Autodesk Fusion 360 part; units mm, degrees
(part 3 of 5)
  line L868 (18.5, -98.5) -> (1.5, -98.5)
  line L869 (1.5, -98.5) -> (1.5, -81.5)
  line L870 (1.5, -81.5) -> (18.5, -81.5)
  line L871 (18.5, -81.5) -> (18.5, -98.5)
  line L872 (38.5, -98.5) -> (21.5, -98.5)
  line L873 (21.5, -98.5) -> (21.5, -81.5)
  line L874 (21.5, -81.5) -> (38.5, -81.5)
  line L875 (38.5, -81.5) -> (38.5, -98.5)
  line L876 (58.5, -98.5) -> (41.5, -98.5)
  line L877 (41.5, -98.5) -> (41.5, -81.5)
  line L878 (41.5, -81.5) -> (58.5, -81.5)
  line L879 (58.5, -81.5) -> (58.5, -98.5)
  line L880 (-105, -220) -> (105, -220)
  line L881 (105, -220) -> (105, 220)
  line L882 (105, 220) -> (-105, 220)
  line L883 (-105, 220) -> (-105, -220)
  line L884 (105, 220) -> (100, 220) construction
  line L885 (-105, 220) -> (-100, 220) construction
  line L886 (-100, 220) -> (-100, -220)
  line L887 (100, 220) -> (100, -220)
  dimension "d16" = 5
  dimension "d17" = 5
  constraint coincident L881.end L882.start
  constraint perpendicular L881 L884
  constraint coincident L882.end L883.start
  constraint perpendicular L883 L885
  constraint coincident L880 L886.end
  constraint perpendicular L880 L886
  constraint coincident L880 L887.end
  constraint perpendicular L880 L887
  measures "d16" distance of L881.end L884.end
  measures "d17" distance of L882.end L885.end
extrude "Extrude4" add sketch "Sketch2" along normal blind 1.6 contours L880 L882 L883 L886 | L880 L881 L882 L887 bodies 1
sketch "Sketch3" plane through (0, 0, 0) normal (0, 0, -1) x (-1, 0, 0)
  line L0 (-100, 220) -> (-100, -220)
  line L1 (-100, -220) -> (100, -220)
  line L2 (100, -220) -> (100, 220)
  line L3 (100, 220) -> (-100, 220)
  line L4 (58.5, -98.5) -> (41.5, -98.5)
  line L5 (41.5, -98.5) -> (41.5, -81.5)
  line L6 (41.5, -81.5) -> (58.5, -81.5)
  line L7 (58.5, -81.5) -> (58.5, -98.5)
  line L8 (38.5, -98.5) -> (21.5, -98.5)
  line L9 (21.5, -98.5) -> (21.5, -81.5)
  line L10 (21.5, -81.5) -> (38.5, -81.5)
  line L11 (38.5, -81.5) -> (38.5, -98.5)
  line L12 (18.5, -98.5) -> (1.5, -98.5)
  line L13 (1.5, -98.5) -> (1.5, -81.5)
  line L14 (1.5, -81.5) -> (18.5, -81.5)
  line L15 (18.5, -81.5) -> (18.5, -98.5)
  line L16 (-1.5, -98.5) -> (-18.5, -98.5)
  line L17 (-18.5, -98.5) -> (-18.5, -81.5)
  line L18 (-18.5, -81.5) -> (-1.5, -81.5)
  line L19 (-1.5, -81.5) -> (-1.5, -98.5)
  line L20 (-21.5, -98.5) -> (-38.5, -98.5)
  line L21 (-38.5, -98.5) -> (-38.5, -81.5)
  line L22 (-38.5, -81.5) -> (-21.5, -81.5)
  line L23 (-21.5, -81.5) -> (-21.5, -98.5)
  line L24 (-41.5, -98.5) -> (-58.5, -98.5)
  line L25 (-58.5, -98.5) -> (-58.5, -81.5)
  line L26 (-58.5, -81.5) -> (-41.5, -81.5)
  line L27 (-41.5, -81.5) -> (-41.5, -98.5)
  line L28 (-61.5, -98.5) -> (-78.5, -98.5)
  line L29 (-78.5, -98.5) -> (-78.5, -81.5)
  line L30 (-78.5, -81.5) -> (-61.5, -81.5)
  line L31 (-61.5, -81.5) -> (-61.5, -98.5)
  line L32 (-81.5, -98.5) -> (-98.5, -98.5)
  line L33 (-98.5, -98.5) -> (-98.5, -81.5)
  line L34 (-98.5, -81.5) -> (-81.5, -81.5)
  line L35 (-81.5, -81.5) -> (-81.5, -98.5)
  line L36 (98.5, -78.5) -> (81.5, -78.5)
  line L37 (81.5, -78.5) -> (81.5, -61.5)
  line L38 (81.5, -61.5) -> (98.5, -61.5)
  line L39 (98.5, -61.5) -> (98.5, -78.5)
  line L40 (78.5, -78.5) -> (61.5, -78.5)
  line L41 (61.5, -78.5) -> (61.5, -61.5)
  line L42 (61.5, -61.5) -> (78.5, -61.5)
  line L43 (78.5, -61.5) -> (78.5, -78.5)
  line L44 (58.5, -78.5) -> (41.5, -78.5)
  line L45 (41.5, -78.5) -> (41.5, -61.5)
  line L46 (41.5, -61.5) -> (58.5, -61.5)
  line L47 (58.5, -61.5) -> (58.5, -78.5)
  line L48 (38.5, -78.5) -> (21.5, -78.5)
  line L49 (21.5, -78.5) -> (21.5, -61.5)
  line L50 (21.5, -61.5) -> (38.5, -61.5)
  line L51 (38.5, -61.5) -> (38.5, -78.5)
  line L52 (18.5, -78.5) -> (1.5, -78.5)
  line L53 (1.5, -78.5) -> (1.5, -61.5)
  line L54 (1.5, -61.5) -> (18.5, -61.5)
  line L55 (18.5, -61.5) -> (18.5, -78.5)
  line L56 (-1.5, -78.5) -> (-18.5, -78.5)
  line L57 (-18.5, -78.5) -> (-18.5, -61.5)
  line L58 (-18.5, -61.5) -> (-1.5, -61.5)
  line L59 (-1.5, -61.5) -> (-1.5, -78.5)
  line L60 (-21.5, -78.5) -> (-38.5, -78.5)
  line L61 (-38.5, -78.5) -> (-38.5, -61.5)
  line L62 (-38.5, -61.5) -> (-21.5, -61.5)
  line L63 (-21.5, -61.5) -> (-21.5, -78.5)
  line L64 (-41.5, -78.5) -> (-58.5, -78.5)
  line L65 (-58.5, -78.5) -> (-58.5, -61.5)
  line L66 (-58.5, -61.5) -> (-41.5, -61.5)
  line L67 (-41.5, -61.5) -> (-41.5, -78.5)
  line L68 (-61.5, -78.5) -> (-78.5, -78.5)
  line L69 (-78.5, -78.5) -> (-78.5, -61.5)
  line L70 (-78.5, -61.5) -> (-61.5, -61.5)
  line L71 (-61.5, -61.5) -> (-61.5, -78.5)
  line L72 (-81.5, -78.5) -> (-98.5, -78.5)
  line L73 (-98.5, -78.5) -> (-98.5, -61.5)
  line L74 (-98.5, -61.5) -> (-81.5, -61.5)
  line L75 (-81.5, -61.5) -> (-81.5, -78.5)
  line L76 (98.5, -58.5) -> (81.5, -58.5)
  line L77 (81.5, -58.5) -> (81.5, -41.5)
  line L78 (81.5, -41.5) -> (98.5, -41.5)
  line L79 (98.5, -41.5) -> (98.5, -58.5)
  line L80 (78.5, -58.5) -> (61.5, -58.5)
  line L81 (61.5, -58.5) -> (61.5, -41.5)
  line L82 (61.5, -41.5) -> (78.5, -41.5)
  line L83 (78.5, -41.5) -> (78.5, -58.5)
  line L84 (58.5, -58.5) -> (41.5, -58.5)
  line L85 (41.5, -58.5) -> (41.5, -41.5)
  line L86 (41.5, -41.5) -> (58.5, -41.5)
  line L87 (58.5, -41.5) -> (58.5, -58.5)
  line L88 (38.5, -58.5) -> (21.5, -58.5)
  line L89 (21.5, -58.5) -> (21.5, -41.5)
  line L90 (21.5, -41.5) -> (38.5, -41.5)
  line L91 (38.5, -41.5) -> (38.5, -58.5)
  line L92 (18.5, -58.5) -> (1.5, -58.5)
  line L93 (1.5, -58.5) -> (1.5, -41.5)
  line L94 (1.5, -41.5) -> (18.5, -41.5)
  line L95 (18.5, -41.5) -> (18.5, -58.5)
  line L96 (-21.5, -58.5) -> (-38.5, -58.5)
  line L97 (-38.5, -58.5) -> (-38.5, -41.5)
  line L98 (-38.5, -41.5) -> (-21.5, -41.5)
  line L99 (-21.5, -41.5) -> (-21.5, -58.5)
  line L100 (78.5, 121.5) -> (61.5, 121.5)
  line L101 (61.5, 121.5) -> (61.5, 138.5)
  line L102 (61.5, 138.5) -> (78.5, 138.5)
  line L103 (78.5, 138.5) -> (78.5, 121.5)
  line L104 (18.5, 161.5) -> (1.5, 161.5)
  line L105 (1.5, 161.5) -> (1.5, 178.5)
  line L106 (1.5, 178.5) -> (18.5, 178.5)
  line L107 (18.5, 178.5) -> (18.5, 161.5)
  line L108 (-1.5, 161.5) -> (-18.5, 161.5)
  line L109 (-18.5, 161.5) -> (-18.5, 178.5)
  line L110 (-18.5, 178.5) -> (-1.5, 178.5)
  line L111 (-1.5, 178.5) -> (-1.5, 161.5)
  line L112 (-21.5, 161.5) -> (-38.5, 161.5)
  line L113 (-38.5, 161.5) -> (-38.5, 178.5)
  line L114 (-38.5, 178.5) -> (-21.5, 178.5)
  line L115 (-21.5, 178.5) -> (-21.5, 161.5)
  line L116 (-41.5, 161.5) -> (-58.5, 161.5)
  line L117 (-58.5, 161.5) -> (-58.5, 178.5)
  line L118 (-58.5, 178.5) -> (-41.5, 178.5)
  line L119 (-41.5, 178.5) -> (-41.5, 161.5)
  line L120 (-61.5, 161.5) -> (-78.5, 161.5)
  line L121 (-78.5, 161.5) -> (-78.5, 178.5)
  line L122 (-78.5, 178.5) -> (-61.5, 178.5)
  line L123 (-61.5, 178.5) -> (-61.5, 161.5)
  line L124 (-81.5, 161.5) -> (-98.5, 161.5)
  line L125 (-98.5, 161.5) -> (-98.5, 178.5)
  line L126 (-98.5, 178.5) -> (-81.5, 178.5)
  line L127 (-81.5, 178.5) -> (-81.5, 161.5)
  line L128 (98.5, 181.5) -> (81.5, 181.5)
  line L129 (81.5, 181.5) -> (81.5, 198.5)
  line L130 (81.5, 198.5) -> (98.5, 198.5)
  line L131 (98.5, 198.5) -> (98.5, 181.5)
  line L132 (78.5, 181.5) -> (61.5, 181.5)
  line L133 (61.5, 181.5) -> (61.5, 198.5)
  line L134 (61.5, 198.5) -> (78.5, 198.5)
  line L135 (78.5, 198.5) -> (78.5, 181.5)
  line L136 (58.5, 181.5) -> (41.5, 181.5)
  line L137 (41.5, 181.5) -> (41.5, 198.5)
  line L138 (41.5, 198.5) -> (58.5, 198.5)
  line L139 (58.5, 198.5) -> (58.5, 181.5)
  line L140 (38.5, 181.5) -> (21.5, 181.5)
  line L141 (21.5, 181.5) -> (21.5, 198.5)
  line L142 (21.5, 198.5) -> (38.5, 198.5)
  line L143 (38.5, 198.5) -> (38.5, 181.5)
  line L144 (18.5, 181.5) -> (1.5, 181.5)
  line L145 (1.5, 181.5) -> (1.5, 198.5)
  line L146 (1.5, 198.5) -> (18.5, 198.5)
  line L147 (18.5, 198.5) -> (18.5, 181.5)
  line L148 (-1.5, 181.5) -> (-18.5, 181.5)
  line L149 (-18.5, 181.5) -> (-18.5, 198.5)
  line L150 (-18.5, 198.5) -> (-1.5, 198.5)
  line L151 (-1.5, 198.5) -> (-1.5, 181.5)
  line L152 (-21.5, 181.5) -> (-38.5, 181.5)
  line L153 (-38.5, 181.5) -> (-38.5, 198.5)
  line L154 (-38.5, 198.5) -> (-21.5, 198.5)
  line L155 (-21.5, 198.5) -> (-21.5, 181.5)
  line L156 (-41.5, 181.5) -> (-58.5, 181.5)
  line L157 (-58.5, 181.5) -> (-58.5, 198.5)
  line L158 (-58.5, 198.5) -> (-41.5, 198.5)
  line L159 (-41.5, 198.5) -> (-41.5, 181.5)
  line L160 (-61.5, 181.5) -> (-78.5, 181.5)
  line L161 (-78.5, 181.5) -> (-78.5, 198.5)
  line L162 (-78.5, 198.5) -> (-61.5, 198.5)
  line L163 (-61.5, 198.5) -> (-61.5, 181.5)
  line L164 (-81.5, 181.5) -> (-98.5, 181.5)
  line L165 (-98.5, 181.5) -> (-98.5, 198.5)
  line L166 (-98.5, 198.5) -> (-81.5, 198.5)
  line L167 (-81.5, 198.5) -> (-81.5, 181.5)
  line L168 (98.5, 201.5) -> (81.5, 201.5)
  line L169 (81.5, 201.5) -> (81.5, 218.5)
  line L170 (81.5, 218.5) -> (98.5, 218.5)
  line L171 (98.5, 218.5) -> (98.5, 201.5)
  line L172 (78.5, 201.5) -> (61.5, 201.5)
  line L173 (61.5, 201.5) -> (61.5, 218.5)
  line L174 (61.5, 218.5) -> (78.5, 218.5)
  line L175 (78.5, 218.5) -> (78.5, 201.5)
  line L176 (58.5, 201.5) -> (41.5, 201.5)
  line L177 (41.5, 201.5) -> (41.5, 218.5)
  line L178 (41.5, 218.5) -> (58.5, 218.5)
  line L179 (58.5, 218.5) -> (58.5, 201.5)
  line L180 (38.5, 201.5) -> (21.5, 201.5)
  line L181 (21.5, 201.5) -> (21.5, 218.5)
  line L182 (21.5, 218.5) -> (38.5, 218.5)
  line L183 (38.5, 218.5) -> (38.5, 201.5)
  line L184 (18.5, 201.5) -> (1.5, 201.5)
  line L185 (1.5, 201.5) -> (1.5, 218.5)
  line L186 (1.5, 218.5) -> (18.5, 218.5)
  line L187 (18.5, 218.5) -> (18.5, 201.5)
  line L188 (-1.5, 201.5) -> (-18.5, 201.5)
  line L189 (-18.5, 201.5) -> (-18.5, 218.5)
  line L190 (-18.5, 218.5) -> (-1.5, 218.5)
  line L191 (-1.5, 218.5) -> (-1.5, 201.5)
  line L192 (-21.5, 201.5) -> (-38.5, 201.5)
  line L193 (-38.5, 201.5) -> (-38.5, 218.5)
  line L194 (-38.5, 218.5) -> (-21.5, 218.5)
  line L195 (-21.5, 218.5) -> (-21.5, 201.5)
  line L196 (-41.5, 201.5) -> (-58.5, 201.5)
  line L197 (-58.5, 201.5) -> (-58.5, 218.5)
  line L198 (-58.5, 218.5) -> (-41.5, 218.5)
  line L199 (-41.5, 218.5) -> (-41.5, 201.5)
  line L200 (-61.5, 201.5) -> (-78.5, 201.5)
  line L201 (-78.5, 201.5) -> (-78.5, 218.5)
  line L202 (-78.5, 218.5) -> (-61.5, 218.5)
  line L203 (-61.5, 218.5) -> (-61.5, 201.5)
  line L204 (-81.5, 201.5) -> (-98.5, 201.5)
  line L205 (-98.5, 201.5) -> (-98.5, 218.5)
  line L206 (-98.5, 218.5) -> (-81.5, 218.5)
  line L207 (-81.5, 218.5) -> (-81.5, 201.5)
  line L208 (-61.5, -58.5) -> (-78.5, -58.5)
  line L209 (-78.5, -58.5) -> (-78.5, -41.5)
  line L210 (-78.5, -41.5) -> (-61.5, -41.5)
  line L211 (-61.5, -41.5) -> (-61.5, -58.5)
  line L212 (-81.5, -58.5) -> (-98.5, -58.5)
  line L213 (-98.5, -58.5) -> (-98.5, -41.5)
  line L214 (-98.5, -41.5) -> (-81.5, -41.5)
  line L215 (-81.5, -41.5) -> (-81.5, -58.5)
  line L216 (98.5, -38.5) -> (81.5, -38.5)
  line L217 (81.5, -38.5) -> (81.5, -21.5)
  line L218 (81.5, -21.5) -> (98.5, -21.5)
  line L219 (98.5, -21.5) -> (98.5, -38.5)
  line L220 (78.5, -38.5) -> (61.5, -38.5)
  line L221 (61.5, -38.5) -> (61.5, -21.5)
  line L222 (61.5, -21.5) -> (78.5, -21.5)
  line L223 (78.5, -21.5) -> (78.5, -38.5)
  line L224 (58.5, -38.5) -> (41.5, -38.5)
  line L225 (41.5, -38.5) -> (41.5, -21.5)
  line L226 (41.5, -21.5) -> (58.5, -21.5)
  line L227 (58.5, -21.5) -> (58.5, -38.5)
  line L228 (38.5, -38.5) -> (21.5, -38.5)
  line L229 (21.5, -38.5) -> (21.5, -21.5)
  line L230 (21.5, -21.5) -> (38.5, -21.5)
  line L231 (38.5, -21.5) -> (38.5, -38.5)
  line L232 (18.5, -38.5) -> (1.5, -38.5)
  line L233 (1.5, -38.5) -> (1.5, -21.5)
  line L234 (1.5, -21.5) -> (18.5, -21.5)
  line L235 (18.5, -21.5) -> (18.5, -38.5)
  line L236 (-1.5, -38.5) -> (-18.5, -38.5)
  line L237 (-18.5, -38.5) -> (-18.5, -21.5)
  line L238 (-18.5, -21.5) -> (-1.5, -21.5)
  line L239 (-1.5, -21.5) -> (-1.5, -38.5)
  line L240 (-21.5, -38.5) -> (-38.5, -38.5)
  line L241 (-38.5, -38.5) -> (-38.5, -21.5)
  line L242 (-38.5, -21.5) -> (-21.5, -21.5)
  line L243 (-21.5, -21.5) -> (-21.5, -38.5)
  line L244 (-41.5, -38.5) -> (-58.5, -38.5)
  line L245 (-58.5, -38.5) -> (-58.5, -21.5)
  line L246 (-58.5, -21.5) -> (-41.5, -21.5)
  line L247 (-41.5, -21.5) -> (-41.5, -38.5)
  line L248 (-61.5, -38.5) -> (-78.5, -38.5)
  line L249 (-78.5, -38.5) -> (-78.5, -21.5)
  line L250 (-78.5, -21.5) -> (-61.5, -21.5)
  line L251 (-61.5, -21.5) -> (-61.5, -38.5)
  line L252 (-81.5, -38.5) -> (-98.5, -38.5)
  line L253 (-98.5, -38.5) -> (-98.5, -21.5)
  line L254 (-98.5, -21.5) -> (-81.5, -21.5)
  line L255 (-81.5, -21.5) -> (-81.5, -38.5)
  line L256 (98.5, -18.5) -> (81.5, -18.5)
  line L257 (81.5, -18.5) -> (81.5, -1.5)
  line L258 (81.5, -1.5) -> (98.5, -1.5)
  line L259 (98.5, -1.5) -> (98.5, -18.5)
  line L260 (78.5, -18.5) -> (61.5, -18.5)
  line L261 (61.5, -18.5) -> (61.5, -1.5)
  line L262 (61.5, -1.5) -> (78.5, -1.5)
  line L263 (78.5, -1.5) -> (78.5, -18.5)
  line L264 (58.5, -18.5) -> (41.5, -18.5)
  line L265 (41.5, -18.5) -> (41.5, -1.5)
  line L266 (41.5, -1.5) -> (58.5, -1.5)
  line L267 (58.5, -1.5) -> (58.5, -18.5)
  line L268 (38.5, -18.5) -> (21.5, -18.5)
  line L269 (21.5, -18.5) -> (21.5, -1.5)
  line L270 (21.5, -1.5) -> (38.5, -1.5)
  line L271 (38.5, -1.5) -> (38.5, -18.5)
  line L272 (18.5, -18.5) -> (1.5, -18.5)
  line L273 (1.5, -18.5) -> (1.5, -1.5)
  line L274 (1.5, -1.5) -> (18.5, -1.5)
  line L275 (18.5, -1.5) -> (18.5, -18.5)
  line L276 (-1.5, -18.5) -> (-18.5, -18.5)
  line L277 (-18.5, -18.5) -> (-18.5, -1.5)
  line L278 (-18.5, -1.5) -> (-1.5, -1.5)
  line L279 (-1.5, -1.5) -> (-1.5, -18.5)
  line L280 (-21.5, -18.5) -> (-38.5, -18.5)
  line L281 (-38.5, -18.5) -> (-38.5, -1.5)
  line L282 (-38.5, -1.5) -> (-21.5, -1.5)
  line L283 (-21.5, -1.5) -> (-21.5, -18.5)
  line L284 (-41.5, -18.5) -> (-58.5, -18.5)
  line L285 (-58.5, -18.5) -> (-58.5, -1.5)
  line L286 (-58.5, -1.5) -> (-41.5, -1.5)
  line L287 (-41.5, -1.5) -> (-41.5, -18.5)
  line L288 (-61.5, -18.5) -> (-78.5, -18.5)
  line L289 (-78.5, -18.5) -> (-78.5, -1.5)
  line L290 (-78.5, -1.5) -> (-61.5, -1.5)
  line L291 (-61.5, -1.5) -> (-61.5, -18.5)
  line L292 (-81.5, -18.5) -> (-98.5, -18.5)
  line L293 (-98.5, -18.5) -> (-98.5, -1.5)
  line L294 (-98.5, -1.5) -> (-81.5, -1.5)
  line L295 (-81.5, -1.5) -> (-81.5, -18.5)
  line L296 (98.5, 1.5) -> (81.5, 1.5)
  line L297 (81.5, 1.5) -> (81.5, 18.5)
  line L298 (81.5, 18.5) -> (98.5, 18.5)
  line L299 (98.5, 18.5) -> (98.5, 1.5)
  line L300 (78.5, 1.5) -> (61.5, 1.5)
  line L301 (61.5, 1.5) -> (61.5, 18.5)
  line L302 (61.5, 18.5) -> (78.5, 18.5)
  line L303 (78.5, 18.5) -> (78.5, 1.5)
  line L304 (58.5, 1.5) -> (41.5, 1.5)
  line L305 (41.5, 1.5) -> (41.5, 18.5)
  line L306 (41.5, 18.5) -> (58.5, 18.5)
  line L307 (58.5, 18.5) -> (58.5, 1.5)
  line L308 (38.5, 1.5) -> (21.5, 1.5)
  line L309 (21.5, 1.5) -> (21.5, 18.5)
  line L310 (21.5, 18.5) -> (38.5, 18.5)
  line L311 (38.5, 18.5) -> (38.5, 1.5)
  line L312 (18.5, 1.5) -> (1.5, 1.5)
  line L313 (1.5, 1.5) -> (1.5, 18.5)
  line L314 (1.5, 18.5) -> (18.5, 18.5)
  line L315 (18.5, 18.5) -> (18.5, 1.5)
  line L316 (-1.5, 1.5) -> (-18.5, 1.5)
  line L317 (-18.5, 1.5) -> (-18.5, 18.5)
  line L318 (-18.5, 18.5) -> (-1.5, 18.5)
  line L319 (-1.5, 18.5) -> (-1.5, 1.5)
  line L320 (-21.5, 1.5) -> (-38.5, 1.5)
  line L321 (-38.5, 1.5) -> (-38.5, 18.5)
  line L322 (-38.5, 18.5) -> (-21.5, 18.5)
  line L323 (-21.5, 18.5) -> (-21.5, 1.5)
  line L324 (-41.5, 1.5) -> (-58.5, 1.5)
  line L325 (-58.5, 1.5) -> (-58.5, 18.5)
  line L326 (-58.5, 18.5) -> (-41.5, 18.5)
  line L327 (-41.5, 18.5) -> (-41.5, 1.5)
  line L328 (-61.5, 1.5) -> (-78.5, 1.5)
  line L329 (-78.5, 1.5) -> (-78.5, 18.5)
  line L330 (-78.5, 18.5) -> (-61.5, 18.5)
  line L331 (-61.5, 18.5) -> (-61.5, 1.5)
  line L332 (-81.5, 1.5) -> (-98.5, 1.5)
  line L333 (-98.5, 1.5) -> (-98.5, 18.5)
  line L334 (-98.5, 18.5) -> (-81.5, 18.5)
  line L335 (-81.5, 18.5) -> (-81.5, 1.5)
  line L336 (98.5, 21.5) -> (81.5, 21.5)
  line L337 (81.5, 21.5) -> (81.5, 38.5)
  line L338 (81.5, 38.5) -> (98.5, 38.5)
  line L339 (98.5, 38.5) -> (98.5, 21.5)
  line L340 (78.5, 21.5) -> (61.5, 21.5)
  line L341 (61.5, 21.5) -> (61.5, 38.5)
  line L342 (61.5, 38.5) -> (78.5, 38.5)
  line L343 (78.5, 38.5) -> (78.5, 21.5)
  line L344 (58.5, 21.5) -> (41.5, 21.5)
  line L345 (41.5, 21.5) -> (41.5, 38.5)
  line L346 (41.5, 38.5) -> (58.5, 38.5)
  line L347 (58.5, 38.5) -> (58.5, 21.5)
  line L348 (38.5, 21.5) -> (21.5, 21.5)
  line L349 (21.5, 21.5) -> (21.5, 38.5)
  line L350 (21.5, 38.5) -> (38.5, 38.5)
  line L351 (38.5, 38.5) -> (38.5, 21.5)
  line L352 (18.5, 21.5) -> (1.5, 21.5)
  line L353 (1.5, 21.5) -> (1.5, 38.5)
  line L354 (1.5, 38.5) -> (18.5, 38.5)
  line L355 (18.5, 38.5) -> (18.5, 21.5)
  line L356 (-1.5, 21.5) -> (-18.5, 21.5)
  line L357 (-18.5, 21.5) -> (-18.5, 38.5)
  line L358 (-18.5, 38.5) -> (-1.5, 38.5)
  line L359 (-1.5, 38.5) -> (-1.5, 21.5)
  line L360 (-21.5, 21.5) -> (-38.5, 21.5)
  line L361 (-38.5, 21.5) -> (-38.5, 38.5)
  line L362 (-38.5, 38.5) -> (-21.5, 38.5)
  line L363 (-21.5, 38.5) -> (-21.5, 21.5)
  line L364 (-41.5, 21.5) -> (-58.5, 21.5)
  line L365 (-58.5, 21.5) -> (-58.5, 38.5)
  line L366 (-58.5, 38.5) -> (-41.5, 38.5)
  line L367 (-41.5, 38.5) -> (-41.5, 21.5)
  line L368 (-61.5, 21.5) -> (-78.5, 21.5)
  line L369 (-78.5, 21.5) -> (-78.5, 38.5)
  line L370 (-78.5, 38.5) -> (-61.5, 38.5)
  line L371 (-61.5, 38.5) -> (-61.5, 21.5)
  line L372 (-81.5, 21.5) -> (-98.5, 21.5)
  line L373 (-98.5, 21.5) -> (-98.5, 38.5)
  line L374 (-98.5, 38.5) -> (-81.5, 38.5)
  line L375 (-81.5, 38.5) -> (-81.5, 21.5)
  line L376 (98.5, 41.5) -> (81.5, 41.5)
  line L377 (81.5, 41.5) -> (81.5, 58.5)
  line L378 (81.5, 58.5) -> (98.5, 58.5)
  line L379 (98.5, 58.5) -> (98.5, 41.5)
  line L380 (78.5, 41.5) -> (61.5, 41.5)
  line L381 (61.5, 41.5) -> (61.5, 58.5)
  line L382 (61.5, 58.5) -> (78.5, 58.5)
  line L383 (78.5, 58.5) -> (78.5, 41.5)
  line L384 (58.5, 41.5) -> (41.5, 41.5)
  line L385 (41.5, 41.5) -> (41.5, 58.5)
  line L386 (41.5, 58.5) -> (58.5, 58.5)
  line L387 (58.5, 58.5) -> (58.5, 41.5)
  line L388 (38.5, 41.5) -> (21.5, 41.5)
  line L389 (21.5, 41.5) -> (21.5, 58.5)
  line L390 (21.5, 58.5) -> (38.5, 58.5)
  line L391 (38.5, 58.5) -> (38.5, 41.5)
  line L392 (18.5, 41.5) -> (1.5, 41.5)
  line L393 (1.5, 41.5) -> (1.5, 58.5)
  line L394 (1.5, 58.5) -> (18.5, 58.5)
  line L395 (18.5, 58.5) -> (18.5, 41.5)
  line L396 (-1.5, 41.5) -> (-18.5, 41.5)
  line L397 (-18.5, 41.5) -> (-18.5, 58.5)
  line L398 (-18.5, 58.5) -> (-1.5, 58.5)
  line L399 (-1.5, 58.5) -> (-1.5, 41.5)
  line L400 (-21.5, 41.5) -> (-38.5, 41.5)
  line L401 (-38.5, 41.5) -> (-38.5, 58.5)
  line L402 (-38.5, 58.5) -> (-21.5, 58.5)
  line L403 (-21.5, 58.5) -> (-21.5, 41.5)
  line L404 (-41.5, 41.5) -> (-58.5, 41.5)
  line L405 (-58.5, 41.5) -> (-58.5, 58.5)
  line L406 (-58.5, 58.5) -> (-41.5, 58.5)
  line L407 (-41.5, 58.5) -> (-41.5, 41.5)
  line L408 (-61.5, 41.5) -> (-78.5, 41.5)
  line L409 (-78.5, 41.5) -> (-78.5, 58.5)
  line L410 (-78.5, 58.5) -> (-61.5, 58.5)
  line L411 (-61.5, 58.5) -> (-61.5, 41.5)
  line L412 (-81.5, 41.5) -> (-98.5, 41.5)
  line L413 (-98.5, 41.5) -> (-98.5, 58.5)
  line L414 (-98.5, 58.5) -> (-81.5, 58.5)
  line L415 (-81.5, 58.5) -> (-81.5, 41.5)
  line L416 (98.5, 61.5) -> (81.5, 61.5)
  line L417 (81.5, 61.5) -> (81.5, 78.5)
  line L418 (81.5, 78.5) -> (98.5, 78.5)
  line L419 (98.5, 78.5) -> (98.5, 61.5)
  line L420 (78.5, 61.5) -> (61.5, 61.5)
  line L421 (61.5, 61.5) -> (61.5, 78.5)
  line L422 (61.5, 78.5) -> (78.5, 78.5)
  line L423 (78.5, 78.5) -> (78.5, 61.5)
  line L424 (58.5, 61.5) -> (41.5, 61.5)
  line L425 (41.5, 61.5) -> (41.5, 78.5)
  line L426 (41.5, 78.5) -> (58.5, 78.5)
  line L427 (58.5, 78.5) -> (58.5, 61.5)
  line L428 (38.5, 61.5) -> (21.5, 61.5)
  line L429 (21.5, 61.5) -> (21.5, 78.5)
  line L430 (21.5, 78.5) -> (38.5, 78.5)
  line L431 (38.5, 78.5) -> (38.5, 61.5)
  line L432 (18.5, 61.5) -> (1.5, 61.5)
  line L433 (1.5, 61.5) -> (1.5, 78.5)
  line L434 (1.5, 78.5) -> (18.5, 78.5)
  line L435 (18.5, 78.5) -> (18.5, 61.5)
  line L436 (-1.5, 61.5) -> (-18.5, 61.5)
  line L437 (-18.5, 61.5) -> (-18.5, 78.5)
  line L438 (-18.5, 78.5) -> (-1.5, 78.5)
  line L439 (-1.5, 78.5) -> (-1.5, 61.5)
  line L440 (-21.5, 61.5) -> (-38.5, 61.5)
  line L441 (-38.5, 61.5) -> (-38.5, 78.5)
  line L442 (-38.5, 78.5) -> (-21.5, 78.5)
  line L443 (-21.5, 78.5) -> (-21.5, 61.5)
  line L444 (-41.5, 61.5) -> (-58.5, 61.5)
  line L445 (-58.5, 61.5) -> (-58.5, 78.5)
  line L446 (-58.5, 78.5) -> (-41.5, 78.5)
  line L447 (-41.5, 78.5) -> (-41.5, 61.5)
  line L448 (-61.5, 61.5) -> (-78.5, 61.5)
  line L449 (-78.5, 61.5) -> (-78.5, 78.5)
  line L450 (-78.5, 78.5) -> (-61.5, 78.5)
  line L451 (-61.5, 78.5) -> (-61.5, 61.5)
  line L452 (-81.5, 61.5) -> (-98.5, 61.5)
  line L453 (-98.5, 61.5) -> (-98.5, 78.5)
  line L454 (-98.5, 78.5) -> (-81.5, 78.5)
  line L455 (-81.5, 78.5) -> (-81.5, 61.5)
  line L456 (98.5, 81.5) -> (81.5, 81.5)
  line L457 (81.5, 81.5) -> (81.5, 98.5)
  line L458 (81.5, 98.5) -> (98.5, 98.5)
  line L459 (98.5, 98.5) -> (98.5, 81.5)
  line L460 (78.5, 81.5) -> (61.5, 81.5)
  line L461 (61.5, 81.5) -> (61.5, 98.5)
  line L462 (61.5, 98.5) -> (78.5, 98.5)
  line L463 (78.5, 98.5) -> (78.5, 81.5)
  line L464 (58.5, 81.5) -> (41.5, 81.5)
  line L465 (41.5, 81.5) -> (41.5, 98.5)
  line L466 (41.5, 98.5) -> (58.5, 98.5)
  line L467 (58.5, 98.5) -> (58.5, 81.5)
  line L468 (38.5, 81.5) -> (21.5, 81.5)
  line L469 (21.5, 81.5) -> (21.5, 98.5)
  line L470 (21.5, 98.5) -> (38.5, 98.5)
  line L471 (38.5, 98.5) -> (38.5, 81.5)
  line L472 (18.5, 81.5) -> (1.5, 81.5)
  line L473 (1.5, 81.5) -> (1.5, 98.5)
  line L474 (1.5, 98.5) -> (18.5, 98.5)
  line L475 (18.5, 98.5) -> (18.5, 81.5)
  line L476 (-1.5, 81.5) -> (-18.5, 81.5)
  line L477 (-18.5, 81.5) -> (-18.5, 98.5)
  line L478 (-18.5, 98.5) -> (-1.5, 98.5)
  line L479 (-1.5, 98.5) -> (-1.5, 81.5)
  line L480 (-21.5, 81.5) -> (-38.5, 81.5)
  line L481 (-38.5, 81.5) -> (-38.5, 98.5)
  line L482 (-38.5, 98.5) -> (-21.5, 98.5)
  line L483 (-21.5, 98.5) -> (-21.5, 81.5)
  line L484 (-41.5, 81.5) -> (-58.5, 81.5)
  line L485 (-58.5, 81.5) -> (-58.5, 98.5)
  line L486 (-58.5, 98.5) -> (-41.5, 98.5)
  line L487 (-41.5, 98.5) -> (-41.5, 81.5)
  line L488 (-61.5, 81.5) -> (-78.5, 81.5)
  line L489 (-78.5, 81.5) -> (-78.5, 98.5)
  line L490 (-78.5, 98.5) -> (-61.5, 98.5)
  line L491 (-61.5, 98.5) -> (-61.5, 81.5)
  line L492 (-81.5, 81.5) -> (-98.5, 81.5)
  line L493 (-98.5, 81.5) -> (-98.5, 98.5)
  line L494 (-98.5, 98.5) -> (-81.5, 98.5)
  line L495 (-81.5, 98.5) -> (-81.5, 81.5)
  line L496 (98.5, 101.5) -> (81.5, 101.5)
  line L497 (81.5, 101.5) -> (81.5, 118.5)
  line L498 (81.5, 118.5) -> (98.5, 118.5)
  line L499 (98.5, 118.5) -> (98.5, 101.5)
  line L500 (78.5, 101.5) -> (61.5, 101.5)
  line L501 (61.5, 101.5) -> (61.5, 118.5)
  line L502 (61.5, 118.5) -> (78.5, 118.5)
  line L503 (78.5, 118.5) -> (78.5, 101.5)
  line L504 (58.5, 101.5) -> (41.5, 101.5)
  line L505 (41.5, 101.5) -> (41.5, 118.5)
  line L506 (41.5, 118.5) -> (58.5, 118.5)
  line L507 (58.5, 118.5) -> (58.5, 101.5)
  line L508 (38.5, 101.5) -> (21.5, 101.5)
  line L509 (21.5, 101.5) -> (21.5, 118.5)
  line L510 (21.5, 118.5) -> (38.5, 118.5)
  line L511 (38.5, 118.5) -> (38.5, 101.5)
  line L512 (18.5, 101.5) -> (1.5, 101.5)
  line L513 (1.5, 101.5) -> (1.5, 118.5)
  line L514 (1.5, 118.5) -> (18.5, 118.5)
  line L515 (18.5, 118.5) -> (18.5, 101.5)
  line L516 (-1.5, 101.5) -> (-18.5, 101.5)
  line L517 (-18.5, 101.5) -> (-18.5, 118.5)
  line L518 (-18.5, 118.5) -> (-1.5, 118.5)
  line L519 (-1.5, 118.5) -> (-1.5, 101.5)
  line L520 (-21.5, 101.5) -> (-38.5, 101.5)
  line L521 (-38.5, 101.5) -> (-38.5, 118.5)
  line L522 (-38.5, 118.5) -> (-21.5, 118.5)
  line L523 (-21.5, 118.5) -> (-21.5, 101.5)
  line L524 (-41.5, 101.5) -> (-58.5, 101.5)
  line L525 (-58.5, 101.5) -> (-58.5, 118.5)
  line L526 (-58.5, 118.5) -> (-41.5, 118.5)
  line L527 (-41.5, 118.5) -> (-41.5, 101.5)
  line L528 (-61.5, 101.5) -> (-78.5, 101.5)
  line L529 (-78.5, 101.5) -> (-78.5, 118.5)
  line L530 (-78.5, 118.5) -> (-61.5, 118.5)
  line L531 (-61.5, 118.5) -> (-61.5, 101.5)
  line L532 (-81.5, 101.5) -> (-98.5, 101.5)
  line L533 (-98.5, 101.5) -> (-98.5, 118.5)
  line L534 (-98.5, 118.5) -> (-81.5, 118.5)
  line L535 (-81.5, 118.5) -> (-81.5, 101.5)
  line L536 (98.5, 121.5) -> (81.5, 121.5)
  line L537 (81.5, 121.5) -> (81.5, 138.5)
  line L538 (81.5, 138.5) -> (98.5, 138.5)
  line L539 (98.5, 138.5) -> (98.5, 121.5)
  line L540 (78.5, -98.5) -> (61.5, -98.5)
  line L541 (61.5, -98.5) -> (61.5, -81.5)
  line L542 (61.5, -81.5) -> (78.5, -81.5)
  line L543 (78.5, -81.5) -> (78.5, -98.5)
  line L544 (38.5, 161.5) -> (21.5, 161.5)
  line L545 (21.5, 161.5) -> (21.5, 178.5)
  line L546 (21.5, 178.5) -> (38.5, 178.5)
  line L547 (38.5, 178.5) -> (38.5, 161.5)
  line L548 (-21.5, -178.5) -> (-38.5, -178.5)
  line L549 (-38.5, -178.5) -> (-38.5, -161.5)
  line L550 (-38.5, -161.5) -> (-21.5, -161.5)
  line L551 (-21.5, -161.5) -> (-21.5, -178.5)
  line L552 (-41.5, -178.5) -> (-58.5, -178.5)
  line L553 (-58.5, -178.5) -> (-58.5, -161.5)
  line L554 (-58.5, -161.5) -> (-41.5, -161.5)
  line L555 (-41.5, -161.5) -> (-41.5, -178.5)
  line L556 (-61.5, -178.5) -> (-78.5, -178.5)
  line L557 (-78.5, -178.5) -> (-78.5, -161.5)
  line L558 (-78.5, -161.5) -> (-61.5, -161.5)
  line L559 (-61.5, -161.5) -> (-61.5, -178.5)
  line L560 (-81.5, -178.5) -> (-98.5, -178.5)
  line L561 (-98.5, -178.5) -> (-98.5, -161.5)
  line L562 (-98.5, -161.5) -> (-81.5, -161.5)
  line L563 (-81.5, -161.5) -> (-81.5, -178.5)
  line L564 (78.5, -158.5) -> (61.5, -158.5)
  line L565 (61.5, -158.5) -> (61.5, -141.5)
  line L566 (61.5, -141.5) -> (78.5, -141.5)
  line L567 (78.5, -141.5) -> (78.5, -158.5)
  line L568 (98.5, -158.5) -> (81.5, -158.5)
  line L569 (81.5, -158.5) -> (81.5, -141.5)
  line L570 (81.5, -141.5) -> (98.5, -141.5)
  line L571 (98.5, -141.5) -> (98.5, -158.5)
  line L572 (-1.5, -178.5) -> (-18.5, -178.5)
  line L573 (-18.5, -178.5) -> (-18.5, -161.5)
  line L574 (-18.5, -161.5) -> (-1.5, -161.5)
  line L575 (-1.5, -161.5) -> (-1.5, -178.5)
  line L576 (18.5, -178.5) -> (1.5, -178.5)
  line L577 (1.5, -178.5) -> (1.5, -161.5)
  line L578 (1.5, -161.5) -> (18.5, -161.5)
  line L579 (18.5, -161.5) -> (18.5, -178.5)
  line L580 (38.5, -178.5) -> (21.5, -178.5)
  line L581 (21.5, -178.5) -> (21.5, -161.5)
  line L582 (21.5, -161.5) -> (38.5, -161.5)
  line L583 (38.5, -161.5) -> (38.5, -178.5)
  line L584 (58.5, -178.5) -> (41.5, -178.5)
  line L585 (41.5, -178.5) -> (41.5, -161.5)
  line L586 (41.5, -161.5) -> (58.5, -161.5)
  line L587 (58.5, -161.5) -> (58.5, -178.5)
  line L588 (78.5, -178.5) -> (61.5, -178.5)
  line L589 (61.5, -178.5) -> (61.5, -161.5)
  line L590 (61.5, -161.5) -> (78.5, -161.5)
  line L591 (78.5, -161.5) -> (78.5, -178.5)
  line L592 (98.5, -178.5) -> (81.5, -178.5)
  line L593 (81.5, -178.5) -> (81.5, -161.5)
  line L594 (81.5, -161.5) -> (98.5, -161.5)
  line L595 (98.5, -161.5) -> (98.5, -178.5)
  line L596 (-81.5, -198.5) -> (-98.5, -198.5)
  line L597 (-98.5, -198.5) -> (-98.5, -181.5)
  line L598 (-98.5, -181.5) -> (-81.5, -181.5)
  line L599 (-81.5, -181.5) -> (-81.5, -198.5)
  line L600 (-61.5, -198.5) -> (-78.5, -198.5)
  line L601 (-78.5, -198.5) -> (-78.5, -181.5)
  line L602 (-78.5, -181.5) -> (-61.5, -181.5)
  line L603 (-61.5, -181.5) -> (-61.5, -198.5)
  line L604 (-41.5, -198.5) -> (-58.5, -198.5)
  line L605 (-58.5, -198.5) -> (-58.5, -181.5)
  line L606 (-58.5, -181.5) -> (-41.5, -181.5)
  line L607 (-41.5, -181.5) -> (-41.5, -198.5)
  line L608 (-21.5, -198.5) -> (-38.5, -198.5)
  line L609 (-38.5, -198.5) -> (-38.5, -181.5)
  line L610 (-38.5, -181.5) -> (-21.5, -181.5)
  line L611 (-21.5, -181.5) -> (-21.5, -198.5)
  line L612 (-1.5, -198.5) -> (-18.5, -198.5)
  line L613 (-18.5, -198.5) -> (-18.5, -181.5)
  line L614 (-18.5, -181.5) -> (-1.5, -181.5)
  line L615 (-1.5, -181.5) -> (-1.5, -198.5)
  line L616 (18.5, -198.5) -> (1.5, -198.5)
  line L617 (1.5, -198.5) -> (1.5, -181.5)
  line L618 (1.5, -181.5) -> (18.5, -181.5)
  line L619 (18.5, -181.5) -> (18.5, -198.5)
  line L620 (38.5, -198.5) -> (21.5, -198.5)
  line L621 (21.5, -198.5) -> (21.5, -181.5)
  line L622 (21.5, -181.5) -> (38.5, -181.5)
  line L623 (38.5, -181.5) -> (38.5, -198.5)
  line L624 (58.5, -198.5) -> (41.5, -198.5)
  line L625 (41.5, -198.5) -> (41.5, -181.5)
  line L626 (41.5, -181.5) -> (58.5, -181.5)
  line L627 (58.5, -181.5) -> (58.5, -198.5)
  line L628 (78.5, -198.5) -> (61.5, -198.5)
  line L629 (61.5, -198.5) -> (61.5, -181.5)
  line L630 (61.5, -181.5) -> (78.5, -181.5)
  line L631 (78.5, -181.5) -> (78.5, -198.5)
  line L632 (98.5, -198.5) -> (81.5, -198.5)
  line L633 (81.5, -198.5) -> (81.5, -181.5)
  line L634 (81.5, -181.5) -> (98.5, -181.5)
  line L635 (98.5, -181.5) -> (98.5, -198.5)
  line L636 (-81.5, -218.5) -> (-98.5, -218.5)
  line L637 (-98.5, -218.5) -> (-98.5, -201.5)
  line L638 (-98.5, -201.5) -> (-81.5, -201.5)
  line L639 (-81.5, -201.5) -> (-81.5, -218.5)
  line L640 (-61.5, -218.5) -> (-78.5, -218.5)
  line L641 (-78.5, -218.5) -> (-78.5, -201.5)
  line L642 (-78.5, -201.5) -> (-61.5, -201.5)
  line L643 (-61.5, -201.5) -> (-61.5, -218.5)
  line L644 (-41.5, -218.5) -> (-58.5, -218.5)
  line L645 (-58.5, -218.5) -> (-58.5, -201.5)
  line L646 (-58.5, -201.5) -> (-41.5, -201.5)
  line L647 (-41.5, -201.5) -> (-41.5, -218.5)
  line L648 (-21.5, -218.5) -> (-38.5, -218.5)
  line L649 (-38.5, -218.5) -> (-38.5, -201.5)
  line L650 (-38.5, -201.5) -> (-21.5, -201.5)
  line L651 (-21.5, -201.5) -> (-21.5, -218.5)
  line L652 (-1.5, -218.5) -> (-18.5, -218.5)
  line L653 (-18.5, -218.5) -> (-18.5, -201.5)
  line L654 (-18.5, -201.5) -> (-1.5, -201.5)
  line L655 (-1.5, -201.5) -> (-1.5, -218.5)
  line L656 (18.5, -218.5) -> (1.5, -218.5)
  line L657 (1.5, -218.5) -> (1.5, -201.5)
  line L658 (1.5, -201.5) -> (18.5, -201.5)
  line L659 (18.5, -201.5) -> (18.5, -218.5)
  line L660 (38.5, -218.5) -> (21.5, -218.5)
  line L661 (21.5, -218.5) -> (21.5, -201.5)
  line L662 (21.5, -201.5) -> (38.5, -201.5)
  line L663 (38.5, -201.5) -> (38.5, -218.5)
  line L664 (58.5, -218.5) -> (41.5, -218.5)
  line L665 (41.5, -218.5) -> (41.5, -201.5)
  line L666 (41.5, -201.5) -> (58.5, -201.5)
  line L667 (58.5, -201.5) -> (58.5, -218.5)
  line L668 (78.5, -218.5) -> (61.5, -218.5)
  line L669 (61.5, -218.5) -> (61.5, -201.5)
  line L670 (61.5, -201.5) -> (78.5, -201.5)
  line L671 (78.5, -201.5) -> (78.5, -218.5)
  line L672 (98.5, -201.5) -> (98.5, -218.5)
  line L673 (98.5, -218.5) -> (81.5, -218.5)
  line L674 (81.5, -218.5) -> (81.5, -201.5)
  line L675 (81.5, -201.5) -> (98.5, -201.5)
  line L676 (-41.5, -58.5) -> (-58.5, -58.5)
  line L677 (-58.5, -58.5) -> (-58.5, -41.5)
  line L678 (-58.5, -41.5) -> (-41.5, -41.5)
  line L679 (-41.5, -41.5) -> (-41.5, -58.5)
  line L680 (58.5, -158.5) -> (41.5, -158.5)
  line L681 (41.5, -158.5) -> (41.5, -141.5)
  line L682 (41.5, -141.5) -> (58.5, -141.5)
  line L683 (58.5, -141.5) -> (58.5, -158.5)
  line L684 (38.5, -158.5) -> (21.5, -158.5)
  line L685 (21.5, -158.5) -> (21.5, -141.5)
  line L686 (21.5, -141.5) -> (38.5, -141.5)
  line L687 (38.5, -141.5) -> (38.5, -158.5)
  line L688 (18.5, -158.5) -> (1.5, -158.5)
  line L689 (1.5, -158.5) -> (1.5, -141.5)
  line L690 (1.5, -141.5) -> (18.5, -141.5)
  line L691 (18.5, -141.5) -> (18.5, -158.5)
  line L692 (-1.5, -158.5) -> (-18.5, -158.5)
  line L693 (-18.5, -158.5) -> (-18.5, -141.5)
  line L694 (-18.5, -141.5) -> (-1.5, -141.5)
  line L695 (-1.5, -141.5) -> (-1.5, -158.5)
  line L696 (-21.5, -158.5) -> (-38.5, -158.5)
  line L697 (-38.5, -158.5) -> (-38.5, -141.5)
  line L698 (-38.5, -141.5) -> (-21.5, -141.5)
  line L699 (-21.5, -141.5) -> (-21.5, -158.5)
  line L700 (-41.5, -158.5) -> (-58.5, -158.5)
  line L701 (-58.5, -158.5) -> (-58.5, -141.5)
  line L702 (-58.5, -141.5) -> (-41.5, -141.5)
  line L703 (-41.5, -141.5) -> (-41.5, -158.5)
  line L704 (-61.5, -158.5) -> (-78.5, -158.5)
  line L705 (-78.5, -158.5) -> (-78.5, -141.5)
  line L706 (-78.5, -141.5) -> (-61.5, -141.5)
  line L707 (-61.5, -141.5) -> (-61.5, -158.5)
  line L708 (-81.5, -158.5) -> (-98.5, -158.5)
  line L709 (-98.5, -158.5) -> (-98.5, -141.5)
  line L710 (-98.5, -141.5) -> (-81.5, -141.5)
  line L711 (-81.5, -141.5) -> (-81.5, -158.5)
  line L712 (98.5, -138.5) -> (81.5, -138.5)
  line L713 (81.5, -138.5) -> (81.5, -121.5)
  line L714 (81.5, -121.5) -> (98.5, -121.5)
  line L715 (98.5, -121.5) -> (98.5, -138.5)
  line L716 (78.5, -138.5) -> (61.5, -138.5)
  line L717 (61.5, -138.5) -> (61.5, -121.5)
  line L718 (61.5, -121.5) -> (78.5, -121.5)
  line L719 (78.5, -121.5) -> (78.5, -138.5)
  line L720 (58.5, -138.5) -> (41.5, -138.5)
  line L721 (41.5, -138.5) -> (41.5, -121.5)
  line L722 (41.5, -121.5) -> (58.5, -121.5)
  line L723 (58.5, -121.5) -> (58.5, -138.5)
  line L724 (38.5, -138.5) -> (21.5, -138.5)
  line L725 (21.5, -138.5) -> (21.5, -121.5)
  line L726 (21.5, -121.5) -> (38.5, -121.5)
  line L727 (38.5, -121.5) -> (38.5, -138.5)
  line L728 (18.5, -138.5) -> (1.5, -138.5)
  line L729 (1.5, -138.5) -> (1.5, -121.5)
  line L730 (1.5, -121.5) -> (18.5, -121.5)
  line L731 (18.5, -121.5) -> (18.5, -138.5)
  line L732 (-1.5, -138.5) -> (-18.5, -138.5)
  line L733 (-18.5, -138.5) -> (-18.5, -121.5)
  line L734 (-18.5, -121.5) -> (-1.5, -121.5)
  line L735 (-1.5, -121.5) -> (-1.5, -138.5)
  line L736 (-21.5, -138.5) -> (-38.5, -138.5)
  line L737 (-38.5, -138.5) -> (-38.5, -121.5)
  line L738 (-38.5, -121.5) -> (-21.5, -121.5)
  line L739 (-21.5, -121.5) -> (-21.5, -138.5)
  line L740 (-41.5, -138.5) -> (-58.5, -138.5)
  line L741 (-58.5, -138.5) -> (-58.5, -121.5)
  line L742 (-58.5, -121.5) -> (-41.5, -121.5)
  line L743 (-41.5, -121.5) -> (-41.5, -138.5)
  line L744 (-61.5, -138.5) -> (-78.5, -138.5)
  line L745 (-78.5, -138.5) -> (-78.5, -121.5)
  line L746 (-78.5, -121.5) -> (-61.5, -121.5)
  line L747 (-61.5, -121.5) -> (-61.5, -138.5)
  line L748 (-81.5, -138.5) -> (-98.5, -138.5)
  line L749 (-98.5, -138.5) -> (-98.5, -121.5)
  line L750 (-98.5, -121.5) -> (-81.5, -121.5)
  line L751 (-81.5, -121.5) -> (-81.5, -138.5)
  line L752 (98.5, -118.5) -> (81.5, -118.5)
  line L753 (81.5, -118.5) -> (81.5, -101.5)
  line L754 (81.5, -101.5) -> (98.5, -101.5)
  line L755 (98.5, -101.5) -> (98.5, -118.5)
  line L756 (78.5, -118.5) -> (61.5, -118.5)
  line L757 (61.5, -118.5) -> (61.5, -101.5)
  line L758 (61.5, -101.5) -> (78.5, -101.5)
  line L759 (78.5, -101.5) -> (78.5, -118.5)
  line L760 (58.5, -118.5) -> (41.5, -118.5)
  line L761 (41.5, -118.5) -> (41.5, -101.5)
  line L762 (41.5, -101.5) -> (58.5, -101.5)
  line L763 (58.5, -101.5) -> (58.5, -118.5)
  line L764 (38.5, -118.5) -> (21.5, -118.5)
  line L765 (21.5, -118.5) -> (21.5, -101.5)
  line L766 (21.5, -101.5) -> (38.5, -101.5)
  line L767 (38.5, -101.5) -> (38.5, -118.5)
  line L768 (18.5, -118.5) -> (1.5, -118.5)
  line L769 (1.5, -118.5) -> (1.5, -101.5)
  line L770 (1.5, -101.5) -> (18.5, -101.5)
  line L771 (18.5, -101.5) -> (18.5, -118.5)
  line L772 (-1.5, -118.5) -> (-18.5, -118.5)
  line L773 (-18.5, -118.5) -> (-18.5, -101.5)
  line L774 (-18.5, -101.5) -> (-1.5, -101.5)
  line L775 (-1.5, -101.5) -> (-1.5, -118.5)
  line L776 (-21.5, -118.5) -> (-38.5, -118.5)
  line L777 (-38.5, -118.5) -> (-38.5, -101.5)
  line L778 (-38.5, -101.5) -> (-21.5, -101.5)
  line L779 (-21.5, -101.5) -> (-21.5, -118.5)
  line L780 (-41.5, -118.5) -> (-58.5, -118.5)
  line L781 (-58.5, -118.5) -> (-58.5, -101.5)
  line L782 (-58.5, -101.5) -> (-41.5, -101.5)
  line L783 (-41.5, -101.5) -> (-41.5, -118.5)
  line L784 (-61.5, -118.5) -> (-78.5, -118.5)
  line L785 (-78.5, -118.5) -> (-78.5, -101.5)
  line L786 (-78.5, -101.5) -> (-61.5, -101.5)
  line L787 (-61.5, -101.5) -> (-61.5, -118.5)
  line L788 (-81.5, -118.5) -> (-98.5, -118.5)
  line L789 (-98.5, -118.5) -> (-98.5, -101.5)
  line L790 (-98.5, -101.5) -> (-81.5, -101.5)
  line L791 (-81.5, -101.5) -> (-81.5, -118.5)
  line L792 (-1.5, -58.5) -> (-18.5, -58.5)
  line L793 (-18.5, -58.5) -> (-18.5, -41.5)
  line L794 (-18.5, -41.5) -> (-1.5, -41.5)
  line L795 (-1.5, -41.5) -> (-1.5, -58.5)
  line L796 (98.5, -98.5) -> (81.5, -98.5)
  line L797 (81.5, -98.5) -> (81.5, -81.5)
  line L798 (81.5, -81.5) -> (98.5, -81.5)
  line L799 (98.5, -81.5) -> (98.5, -98.5)
  line L800 (58.5, 121.5) -> (41.5, 121.5)
  line L801 (41.5, 121.5) -> (41.5, 138.5)
  line L802 (41.5, 138.5) -> (58.5, 138.5)
  line L803 (58.5, 138.5) -> (58.5, 121.5)
  line L804 (58.5, 161.5) -> (41.5, 161.5)
  line L805 (41.5, 161.5) -> (41.5, 178.5)
  line L806 (41.5, 178.5) -> (58.5, 178.5)
  line L807 (58.5, 178.5) -> (58.5, 161.5)
  line L808 (78.5, 161.5) -> (61.5, 161.5)
  line L809 (61.5, 161.5) -> (61.5, 178.5)
  line L810 (61.5, 178.5) -> (78.5, 178.5)
  line L811 (78.5, 178.5) -> (78.5, 161.5)
  line L812 (98.5, 161.5) -> (81.5, 161.5)
  line L813 (81.5, 161.5) -> (81.5, 178.5)
  line L814 (81.5, 178.5) -> (98.5, 178.5)
  line L815 (98.5, 178.5) -> (98.5, 161.5)
  line L816 (-81.5, 141.5) -> (-98.5, 141.5)
  line L817 (-98.5, 141.5) -> (-98.5, 158.5)
  line L818 (-98.5, 158.5) -> (-81.5, 158.5)
  line L819 (-81.5, 158.5) -> (-81.5, 141.5)
  line L820 (-61.5, 141.5) -> (-78.5, 141.5)
  line L821 (-78.5, 141.5) -> (-78.5, 158.5)
  line L822 (-78.5, 158.5) -> (-61.5, 158.5)
  line L823 (-61.5, 158.5) -> (-61.5, 141.5)
  line L824 (-41.5, 141.5) -> (-58.5, 141.5)
  line L825 (-58.5, 141.5) -> (-58.5, 158.5)
  line L826 (-58.5, 158.5) -> (-41.5, 158.5)
  line L827 (-41.5, 158.5) -> (-41.5, 141.5)
  line L828 (-21.5, 141.5) -> (-38.5, 141.5)
  line L829 (-38.5, 141.5) -> (-38.5, 158.5)
  line L830 (-38.5, 158.5) -> (-21.5, 158.5)
  line L831 (-21.5, 158.5) -> (-21.5, 141.5)
  line L832 (-1.5, 141.5) -> (-18.5, 141.5)
  line L833 (-18.5, 141.5) -> (-18.5, 158.5)
  line L834 (-18.5, 158.5) -> (-1.5, 158.5)
  line L835 (-1.5, 158.5) -> (-1.5, 141.5)
  line L836 (18.5, 141.5) -> (1.5, 141.5)
  line L837 (1.5, 141.5) -> (1.5, 158.5)
  line L838 (1.5, 158.5) -> (18.5, 158.5)
  line L839 (18.5, 158.5) -> (18.5, 141.5)
  line L840 (38.5, 141.5) -> (21.5, 141.5)
  line L841 (21.5, 141.5) -> (21.5, 158.5)
  line L842 (21.5, 158.5) -> (38.5, 158.5)
  line L843 (38.5, 158.5) -> (38.5, 141.5)
  line L844 (58.5, 141.5) -> (41.5, 141.5)
  line L845 (41.5, 141.5) -> (41.5, 158.5)
  line L846 (41.5, 158.5) -> (58.5, 158.5)
  line L847 (58.5, 158.5) -> (58.5, 141.5)
  line L848 (78.5, 141.5) -> (61.5, 141.5)
  line L849 (61.5, 141.5) -> (61.5, 158.5)
  line L850 (61.5, 158.5) -> (78.5, 158.5)
  line L851 (78.5, 158.5) -> (78.5, 141.5)
  line L852 (98.5, 141.5) -> (81.5, 141.5)
  line L853 (81.5, 141.5) -> (81.5, 158.5)
  line L854 (81.5, 158.5) -> (98.5, 158.5)
  line L855 (98.5, 158.5) -> (98.5, 141.5)
  line L856 (-81.5, 121.5) -> (-98.5, 121.5)
  line L857 (-98.5, 121.5) -> (-98.5, 138.5)
  line L858 (-98.5, 138.5) -> (-81.5, 138.5)
  line L859 (-81.5, 138.5) -> (-81.5, 121.5)
  line L860 (-61.5, 121.5) -> (-78.5, 121.5)
  line L861 (-78.5, 121.5) -> (-78.5, 138.5)
  line L862 (-78.5, 138.5) -> (-61.5, 138.5)
  line L863 (-61.5, 138.5) -> (-61.5, 121.5)
  line L864 (-41.5, 121.5) -> (-58.5, 121.5)
  line L865 (-58.5, 121.5) -> (-58.5, 138.5)
  line L866 (-58.5, 138.5) -> (-41.5, 138.5)
  line L867 (-41.5, 138.5) -> (-41.5, 121.5)
  line L868 (-21.5, 121.5) -> (-38.5, 121.5)
  line L869 (-38.5, 121.5) -> (-38.5, 138.5)
  line L870 (-38.5, 138.5) -> (-21.5, 138.5)
  line L871 (-21.5, 138.5) -> (-21.5, 121.5)
  line L872 (-1.5, 121.5) -> (-18.5, 121.5)
  line L873 (-18.5, 121.5) -> (-18.5, 138.5)
  line L874 (-18.5, 138.5) -> (-1.5, 138.5)
  line L875 (-1.5, 138.5) -> (-1.5, 121.5)
  line L876 (18.5, 121.5) -> (1.5, 121.5)
  line L877 (1.5, 121.5) -> (1.5, 138.5)
  line L878 (1.5, 138.5) -> (18.5, 138.5)
  line L879 (18.5, 138.5) -> (18.5, 121.5)
  line L880 (38.5, 121.5) -> (21.5, 121.5)
  line L881 (21.5, 121.5) -> (21.5, 138.5)
  line L882 (21.5, 138.5) -> (38.5, 138.5)
  line L883 (38.5, 138.5) -> (38.5, 121.5)
  line L884 (-100, -220) -> (-100, -200) construction
  circle A0 centre (-100, -200) radius 2
  circle A1 centre (-100, -160) radius 2
  circle A2 centre (-100, -120) radius 2
  circle A3 centre (-100, -80) radius 2
  circle A4 centre (-100, -40) radius 2
  circle A5 centre (-100, 0) radius 2
  circle A6 centre (-100, 40) radius 2
  circle A7 centre (-100, 80) radius 2
  circle A8 centre (-100, 120) radius 2
  circle A9 centre (-100, 160) radius 2
  circle A10 centre (-100, 200) radius 2
  dimension "d20" = 20
  dimension "d21" = 4
  dimension "d24" = -400
  dimension "d25" = 0
  constraint coincident L0.end L1.start
  constraint perpendicular L638 L884
  constraint coincident L884.end A0.centre
  measures "d20" distance of L0.end L884.end
  measures "d21" diameter of A0
extrude "Extrude5" add sketch "Sketch3" along normal blind 1.6 contours L0 A10 | L0 A9 | L0 A0 | L0 A8 | L0 A1 | L0 A7 | L0 A2 | L0 A6 | L0 A3 | L0 A5 | L0 A4 picked at (-99.7231, 200.6064) picked at (-99.7231, 160.6064) picked at (-98.4872, -200.1878) picked at (-99.3603, 119.8122) picked at (-98.4872, -160.1878) picked at (-99.3603, 79.8122) picked at (-99.3603, -120.1878) picked at (-99.3603, 39.8122) picked at (-99.3603, -80.1878) picked at (-99.3603, -0.1878) picked at (-99.3603, -40.1878) bodies 1